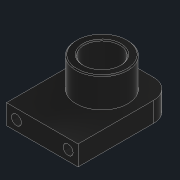
# Autodesk Inventor part: cable_holder
Saved by Autodesk Inventor 2022 (Build 260153000, 153)
## iProperties
Created: 2021-07-24
Part Number: cable_holder
Material: ABS プラスチック
Document SubType Name: Modeling
Designer: yuta0
Density: 1.06 g/cm^3
Appearance: 滑らか - 黒
購入先: 印刷
在庫数: 0.0
Author: yuta0
Autodesk Inventor part; units mm, degrees
ref_plane "YZ Plane" through (0, 0, 0) normal (1, 0, 0) x (0, 1, 0)
ref_plane "XZ Plane" through (0, 0, 0) normal (0, 1, 0) x (-1, 0, 0)
ref_plane "XY Plane" through (0, 0, 0) normal (0, 0, 1) x (1, 0, 0)
sketch "スケッチ1" plane through (0, 0, 0) normal (0, 1, 0) x (-1, 0, 0)
  circle A0 centre (0, 0) radius 9
  line L0 (18, 10) -> (-18, 10)
  line L1 (-18, 10) -> (-18, -18)
  line L2 (-18, -18) -> (18, -18)
  line L3 (18, -18) -> (18, 10)
  line L4 (18, 30) -> (-18, 30)
  line L5 (-18, 30) -> (-18, 10)
  line L6 (-18, 10) -> (18, 10)
  line L7 (18, 10) -> (18, 30)
  line L8 (18, 30) -> (-18, 10) construction
  line L9 (-18, 30) -> (18, 10) construction
  point P0 (0, 20)
  point P1 (0, 20)
  point P2 (20, 10)
  point P3 (-6.6332, 10)
  point P4 (6.6332, 10)
  dimension "d0" = 18
  dimension "d18" = 10
  dimension "d33" = 30
  dimension "d34" = 36
  dimension "d36" = 18
  constraints: 21 end point, 4 parallel, 3 coincident, 3 midpoint, 2 horizontal, 2 perpendicular, 1 centre point, 1 vertical alignment
  measures "d0" diameter of A0
  measures "d18" distance from line of A0.centre L0
  measures "d33" distance from line of point (0, 0) L4
  measures "d34" distance of L4.start L4.end
  measures "d36" distance from line of L2 A0.centre
extrude "押し出し1" add sketch "スケッチ1" along normal mid plane 10
sketch "スケッチ2" plane through (-38, 5, 30) normal (0, 0, 1) x (1, 0, 0)
  line L0 (20, -10) -> (20, 0) projected
  line L1 (56, -10) -> (20, -10) projected
  line L2 (56, 0) -> (56, -10) projected
  point P0 (38, -5)
  point P1 (25, -5)
  point P2 (51, -5)
  dimension "d37" = 5
  dimension "d38" = 5
  dimension "d39" = 5
  constraints: 1 horizontal alignment
  measures "d37" distance from line of L0 point (25, -5)
  measures "d38" distance from line of L1 point (25, -5)
  measures "d39" distance from line of L2 point (51, -5)
hole "穴1" at (-13, 0, 30) at (13, 0, 30) direction (0, 0, -1) diameter 5 depth 6 tip angle 118
fillet "フィレット1" radius 10 2 edges at (18, 0, -18) (-18, 0, -18)
sketch "スケッチ4" plane through (0, 5, 0) normal (0, 1, 0) x (1, 0, 0)
  circle A0 centre (0, 0) radius 13
  circle A1 centre (0, 0) radius 9 projected
  dimension "d43" = 26
  constraints: 1 centre point, 1 coincident
  measures "d43" diameter of A0
extrude "押し出し3" add sketch "スケッチ4" along normal blind 15
chamfer "面取り3" distance 0.5 angle 45 2 edges at (-9, 20, 0) (-13, 20, 0)
